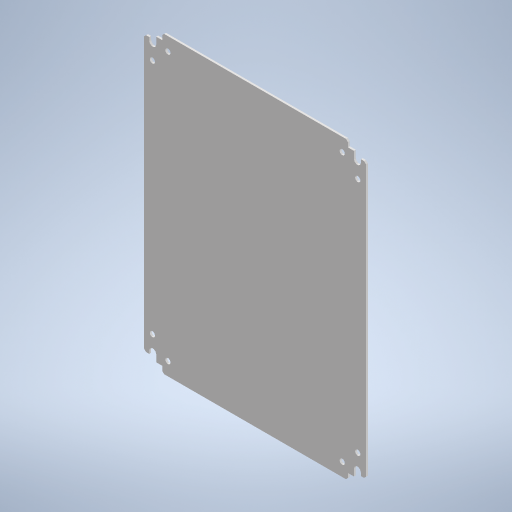
# Autodesk Inventor part: assembly-board
Saved by Autodesk Inventor 2023 (Build 270158030, 158C)
## iProperties
Created: 2024-03-20
Part Number: assembly-board
Material: Generic
Document SubType Name: Modeling
Designer: Imogen Heard
Density: 1 g/cm^3
Appearance: Default
Author: Imogen Heard
Autodesk Inventor part; units mm, degrees
ref_plane "YZ Plane" through (0, 0, 0) normal (1, 0, 0) x (0, 1, 0)
ref_plane "XZ Plane" through (0, 0, 0) normal (0, 1, 0) x (-1, 0, 0)
ref_plane "XY Plane" through (0, 0, 0) normal (0, 0, 1) x (1, 0, 0)
sketch "Sketch1" plane through (0, 0, 0) normal (0, 0, 1) x (1, 0, 0)
  line L0 (-175, 232.5) -> (175, 232.5)
  line L1 (175, 232.5) -> (175, -232.5)
  line L2 (175, -232.5) -> (-175, -232.5)
  line L3 (-175, -232.5) -> (-175, 232.5)
  point P0 (0, 0)
  dimension "d0" = 350
  dimension "d1" = 465
  dimension "d2" = 232.5
  dimension "d3" = 175
  constraints: 8 end point, 2 parallel, 1 horizontal, 1 perpendicular
  measures "d0" distance between parallel lines of L1 L3
  measures "d1" distance between parallel lines of L2 L0
  measures "d2" distance from line of point (0, 0) L0
  measures "d3" distance from line of point (0, 0) L1
extrude "Extrusion1" add sketch "Sketch1" along normal blind 3
sketch "Sketch3" plane through (0, 0, 3) normal (0, 0, 1) x (1, 0, 0)
  line L0 (-175, -232.5) -> (175, -232.5) projected
  line L1 (175, 232.5) -> (-175, 232.5) projected
  line L2 (175, -232.5) -> (175, 232.5) projected
  line L3 (-175, 232.5) -> (-175, -232.5) projected
  line L4 (-175, 232.5) -> (-146.5, 232.5)
  line L5 (-146.5, 232.5) -> (-146.5, 222.5)
  line L6 (-146.5, 222.5) -> (-175, 222.5)
  line L7 (-175, 222.5) -> (-175, 232.5)
  line L8 (-156, 216.5) -> (-175, 216.5)
  line L9 (-175, 216.5) -> (-175, 222.5)
  line L10 (-175, 222.5) -> (-156, 222.5)
  line L11 (-156, 222.5) -> (-156, 216.5)
  line L12 (-156, 216.5) -> (-167, 216.5)
  line L13 (-167, 216.5) -> (-167, 211.5)
  line L14 (-167, 211.5) -> (-156, 211.5)
  line L15 (-156, 211.5) -> (-156, 216.5)
  arc A0 (-167, 211.5) -> (-156, 211.5) centre (-161.5, 211.5) ccw
  line L16 (-146.5, 229.5) -> (-143.5, 232.5)
  line L17 (-175, 213.5) -> (-172, 216.5)
  circle A1 centre (-162, 187) radius 4.2
  circle A2 centre (-137.5, 211.5) radius 4.2
  point P0 (0, 0)
  dimension "d7" = 465
  dimension "d8" = 350
  dimension "d9" = 28.5
  dimension "d10" = 10
  dimension "d11" = 6
  dimension "d12" = 19
  dimension "d14" = 5
  dimension "d15" = 11
  dimension "d16" = 45
  dimension "d17" = 3
  dimension "d18" = 3
  dimension "d19" = 45
  dimension "d22" = 8.4
  dimension "d23" = 13
  dimension "d24" = 13.5
  dimension "d25" = 45.5
  dimension "d26" = 37.5
  dimension "d27" = 21
  constraints: 28 end point, 6 parallel, 3 centre point, 3 horizontal, 3 perpendicular, 3 point on line, 2 coincident, 2 point on circle, 1 equal radius, 1 horizontal alignment, 1 midpoint
  measures "d7" distance between parallel lines of L0 L1
  measures "d8" distance between parallel lines of L2 L3
  measures "d9" distance between parallel lines of L3 L5
  measures "d10" distance between parallel lines of L6 L1
  measures "d11" distance between parallel lines of L8 L6
  measures "d12" distance between parallel lines of L3 L11
  measures "d14" distance between parallel lines of L14 L12
  measures "d15" distance between parallel lines of L13 L15
  measures "d16" angle of L5 L16
  measures "d17" distance of L4.end L16.end
  measures "d18" distance from line of L3 L17.end
  measures "d19" angle of L8 L17
  measures "d22" diameter of A2
  measures "d23" distance from line of L3 A1.centre
  measures "d24" distance from line of L3 A0.centre
  measures "d25" distance from line of A1.centre L1
  measures "d26" distance from line of A2.centre L3
  measures "d27" distance from line of L1 A2.centre
extrude "Extrusion2" cut sketch "Sketch3" against normal through all contours L3 L8 L17 | L3 L6 L11 L8 | L16 L5 L1 | L3 L1 L5 L6 | L8 L15 L14 L13 | L14 A0 | A1 | A2
mirror "Mirror1" about plane through (0, 0, 0) normal (1, 0, 0) of "Extrusion2"
mirror "Mirror2" about plane through (0, 0, 0) normal (0, 1, 0) of "Extrusion2", "Mirror1"
equation "\"d2\" = 0.5 * d1"
equation "\"d3\" = 0.5 * d0"
body "Solid1"
